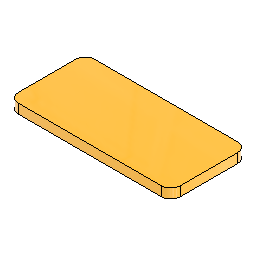
splitboard left v11 (Autodesk Fusion 360 archive; units mm, degrees)
design "battery"
Autodesk Fusion 360 part; units mm, degrees
sketch "Sketch1" plane through (0, 0, 0) normal (0, 0, 1) x (1, 0, 0)
  line L0 (5, 0) -> (80, 0)
  line L1 (85, 5) -> (85, 35)
  line L2 (80, 40) -> (5, 40)
  line L3 (0, 35) -> (0, 5)
  arc A0 (5, 40) -> (0, 35) centre (5, 35) ccw
  arc A1 (0, 5) -> (5, 0) centre (5, 5) ccw
  arc A2 (80, 0) -> (85, 5) centre (80, 5) ccw
  arc A3 (85, 35) -> (80, 40) centre (80, 35) ccw
  point P0 (85, 0)
  point P1 (0, 40)
  dimension "d1" = 85
  dimension "d2" = 40
  dimension "d3" = 5
  constraint horizontal L0
  constraint vertical L1
  constraint horizontal L2
  constraint vertical L3
  constraint coincident P1 L2
  constraint coincident P1 L3
  constraint tangent L2 A0
  constraint tangent L3 A0
  constraint coincident origin L0
  constraint coincident origin L3
  constraint tangent L0 A1
  constraint tangent L3 A1
  constraint equal A0 A1
  constraint coincident P0 L0
  constraint coincident P0 L1
  constraint tangent L0 A2
  constraint tangent L1 A2
  constraint equal A0 A2
  constraint tangent L1 A3
  constraint tangent L2 A3
  constraint equal A0 A3
  measures "d1" distance of origin P0
  measures "d2" distance of origin P1
  measures "d3" radius of A0
extrude "Extrude1" add sketch "Sketch1" along normal blind 5
